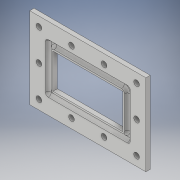
# Autodesk Inventor part: Acrylic Front
Saved by Autodesk Inventor 2018 (Build 220112000, 112)
## iProperties
Created: 2018-04-18
Part Number: Acrylic Front
Material: Generic
Document SubType Name: Modeling
Designer: trent
Density: 1 g/cm^3
Appearance: Default
Author: trent
Autodesk Inventor part; units mm, degrees
ref_plane "YZ Plane" through (0, 0, 0) normal (1, 0, 0) x (0, 1, 0)
ref_plane "XZ Plane" through (0, 0, 0) normal (0, 1, 0) x (-1, 0, 0)
ref_plane "XY Plane" through (0, 0, 0) normal (0, 0, 1) x (1, 0, 0)
sketch "Sketch1" plane through (0, 0, 0) normal (0, 0, 1) x (1, 0, 0)
  line L0 (0, 0) -> (127, 0)
  line L1 (127, 0) -> (127, 88.9)
  line L2 (127, 88.9) -> (0, 88.9)
  line L3 (0, 88.9) -> (0, 0)
  circle A0 centre (10.16, 78.74) radius 3.0988
  circle A1 centre (10.16, 44.45) radius 3.0988
  circle A2 centre (10.16, 10.16) radius 3.0988
  circle A3 centre (45.72, 10.16) radius 3.0988
  circle A4 centre (116.84, 10.16) radius 3.0988
  circle A5 centre (116.84, 44.45) radius 3.0988
  circle A6 centre (116.84, 78.74) radius 3.0988
  circle A7 centre (45.72, 78.74) radius 3.0988
  line L4 (25.4, 25.4) -> (101.6, 25.4)
  line L5 (101.6, 25.4) -> (101.6, 63.5)
  line L6 (101.6, 63.5) -> (25.4, 63.5)
  line L7 (25.4, 63.5) -> (25.4, 25.4)
  line L8 (25.4, 25.4) -> (101.6, 63.5) construction
  line L9 (101.6, 25.4) -> (25.4, 63.5) construction
  circle A8 centre (81.28, 10.16) radius 3.0988
  circle A9 centre (81.28, 78.74) radius 3.0988
  point P0 (63.5, 44.45)
  dimension "d0" = 127
  dimension "d1" = 88.9
  dimension "d3" = 6.1976
  dimension "d4" = 10.16
  dimension "d5" = 10.16
  dimension "d6" = 10.16
  dimension "d7" = 10.16
  dimension "d8" = 44.45
  dimension "d10" = 10.16
  dimension "d11" = 10.16
  dimension "d12" = 10.16
  dimension "d13" = 10.16
  dimension "d14" = 44.45
  dimension "d15" = 10.16
  dimension "d16" = 10.16
  dimension "d17" = 10.16
  dimension "d18" = 10.16
  dimension "d31" = 76.2
  dimension "d32" = 38.1
  dimension "d33" = 44.45
  dimension "d34" = 63.5
  dimension "d42" = 35.56
  dimension "d43" = 35.56
  dimension "d44" = 35.56
  dimension "d46" = 35.56
  dimension "d47" = 35.56
  dimension "d49" = 35.56
  constraints: 20 end point, 10 centre point, 9 equal radius, 4 parallel, 2 horizontal, 2 midpoint, 2 perpendicular
  measures "d0" distance of L2.end L1.end
  measures "d1" distance of L1.end L0.end
  measures "d3" diameter of A0
  measures "d4" distance from line of L2 A0.centre
  measures "d5" distance from line of L3 A0.centre
  measures "d6" distance from line of L3 A2.centre
  measures "d7" distance from line of L0 A2.centre
  measures "d8" distance from line of L0 A1.centre
  measures "d10" distance from line of L2 A7.centre
  measures "d11" distance from line of L3 A1.centre
  measures "d12" distance from line of L2 A6.centre
  measures "d13" distance from line of L1 A6.centre
  measures "d14" distance from line of L0 A5.centre
  measures "d15" distance from line of L1 A5.centre
  measures "d16" distance from line of L0 A4.centre
  measures "d17" distance from line of L1 A4.centre
  measures "d18" distance from line of L0 A3.centre
  measures "d31" distance of L6.end L5.end
  measures "d32" distance of L5.end L4.end
  measures "d33" distance from line of L0 point (63.5, 44.45)
  measures "d34" distance from line of L1 point (63.5, 44.45)
  measures "d42" distance of A0.centre A7.centre
  measures "d43" distance of A7.centre A9.centre
  measures "d44" distance of A6.centre A9.centre
  measures "d46" distance of A8.centre A3.centre
  measures "d47" distance of A2.centre A3.centre
  measures "d49" distance of A4.centre A8.centre
extrude "Extrusion1" add sketch "Sketch1" along normal blind 4.7625
sketch "Sketch3" plane through (0, 0, 4.7625) normal (0, 0, 1) x (1, 0, 0)
  line L0 (25.4, 25.4) -> (25.4, 63.5) projected
  line L1 (25.4, 63.5) -> (101.6, 63.5) projected
  line L2 (101.6, 63.5) -> (101.6, 25.4) projected
  line L3 (101.6, 25.4) -> (25.4, 25.4) projected
  circle A0 centre (45.72, 78.74) radius 3.0988 projected
  circle A1 centre (116.84, 78.74) radius 3.0988 projected
  circle A2 centre (116.84, 44.45) radius 3.0988 projected
  circle A3 centre (116.84, 10.16) radius 3.0988 projected
  circle A4 centre (45.72, 10.16) radius 3.0988 projected
  circle A5 centre (10.16, 10.16) radius 3.0988 projected
  circle A6 centre (10.16, 44.45) radius 3.0988 projected
  circle A7 centre (10.16, 78.74) radius 3.0988 projected
  line L4 (0, 0) -> (127, 0) projected
  line L5 (127, 0) -> (127, 88.9) projected
  line L6 (127, 88.9) -> (0, 88.9) projected
  line L7 (0, 88.9) -> (0, 0) projected
  line L8 (23.495, 62.23) -> (23.495, 26.67)
  line L9 (26.67, 23.495) -> (100.33, 23.495)
  line L10 (103.505, 26.67) -> (103.505, 62.23)
  line L11 (100.33, 65.405) -> (26.67, 65.405)
  line L12 (17.145, 20.32) -> (17.145, 68.58)
  line L13 (20.32, 71.755) -> (106.68, 71.755)
  line L14 (109.855, 68.58) -> (109.855, 20.32)
  line L15 (106.68, 17.145) -> (20.32, 17.145)
  arc A8 (20.32, 71.755) -> (17.145, 68.58) centre (20.32, 68.58) ccw
  arc A9 (26.67, 65.405) -> (23.495, 62.23) centre (26.67, 62.23) ccw
  arc A10 (109.855, 68.58) -> (106.68, 71.755) centre (106.68, 68.58) ccw
  arc A11 (103.505, 62.23) -> (100.33, 65.405) centre (100.33, 62.23) ccw
  arc A12 (100.33, 23.495) -> (103.505, 26.67) centre (100.33, 26.67) ccw
  arc A13 (106.68, 17.145) -> (109.855, 20.32) centre (106.68, 20.32) ccw
  arc A14 (17.145, 20.32) -> (20.32, 17.145) centre (20.32, 20.32) ccw
  arc A15 (23.495, 26.67) -> (26.67, 23.495) centre (26.67, 26.67) ccw
  dimension "d36" = 1.905
  dimension "d37" = 6.35
  dimension "d38" = 3.175
  constraints: 16 end point, 16 point on circle, 16 tangent, 8 centre point, 7 equal radius, 6 other
  measures "d36" distance between parallel lines of L0 L8
  measures "d37" distance between parallel lines of L8 L12
  measures "d38" radius of A8
extrude "Extrusion3" cut sketch "Sketch3" against normal blind 3.175 contours L12 A8 L13 A10 L14 A13 L15 A14
fillet "Fillet2" radius 3.175 16 edges at (18.0749, 70.8251, 1.5875) (63.5, 71.755, 1.5875) (108.9251, 70.8251, 1.5875) (109.855, 44.45, 1.5875) (108.9251, 18.0749, 1.5875) (63.5, 17.145, 1.5875) (18.0749, 18.0749, 1.5875) (17.145, 44.45, 1.5875) (102.5751, 64.4751, 1.5875) (63.5, 65.405, 1.5875) (24.4249, 64.4751, 1.5875) (23.495, 44.45, 1.5875) (24.4249, 24.4249, 1.5875) (63.5, 23.495, 1.5875) (102.5751, 24.4249, 1.5875) (103.505, 44.45, 1.5875)
equation "\"d6\" = d5"
equation "\"d7\" = d4"
equation "\"d8\" = 0.5 * d1"
equation "\"d10\" = d4"
equation "\"d11\" = d5"
equation "\"d12\" = d4"
equation "\"d13\" = d5"
equation "\"d14\" = 0.5 * d1"
equation "\"d15\" = d13"
equation "\"d16\" = d12"
equation "\"d17\" = d13"
equation "\"d18\" = d16"
equation "\"d33\" = 0.5 * d1"
equation "\"d34\" = 0.5 * d0"
equation "\"d43\" = d42"
equation "\"d44\" = d43"
equation "\"d46\" = d42"
equation "\"d47\" = d46"
equation "\"d49\" = d46"
body "Solid1"
